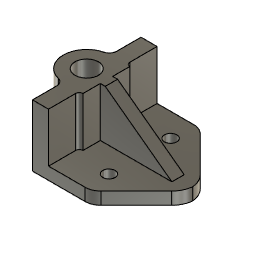
A3 (Autodesk Fusion 360 design; units mm, degrees)
Autodesk Fusion 360 part; units mm, degrees
sketch "Sketch1" plane through (0, 0, 0) normal (0, 0, 1) x (1, 0, 0)
  line L0 (-0.3848, 44) -> (-43, 44)
  line L1 (-43, 44) -> (-43, -44)
  line L2 (-43, -44) -> (-0.3848, -44)
  line L3 (43, 1.8701) -> (43, -1.8701)
  line L4 (37.435, 11.565) -> (8.8076, 40.1924)
  line L5 (37.435, -11.565) -> (8.8076, -40.1924)
  arc A0 (43, -1.8701) -> (37.435, 11.565) centre (24, -1.8701) ccw
  arc A1 (37.435, -11.565) -> (43, 1.8701) centre (24, 1.8701) ccw
  arc A2 (-0.3848, -44) -> (8.8076, -40.1924) centre (-0.3848, -31) ccw
  arc A3 (8.8076, 40.1924) -> (-0.3848, 44) centre (-0.3848, 31) ccw
  point P0 (43, 6)
  point P1 (5, 44)
  point P2 (43, -6)
  point P3 (5, -44)
  dimension "d2" = 88
  dimension "d7" = 19
  dimension "d8" = 19
  dimension "d9" = 13
  dimension "d10" = 13
  constraint horizontal L0
  constraint perpendicular L0 L1
  constraint parallel L0 L2
  constraint parallel L1 L3
  constraint coincident P0 L4
  constraint coincident L3 P0
  constraint tangent L4 A0
  constraint tangent L3 A0
  constraint coincident P2 L5
  constraint coincident L3 P2
  constraint tangent L5 A1
  constraint tangent L3 A1
  constraint coincident P3 L5
  constraint coincident L2 P3
  constraint tangent L5 A2
  constraint tangent L2 A2
  constraint coincident P1 L4
  constraint coincident L0 P1
  constraint tangent L4 A3
  constraint tangent L0 A3
  measures "d2" distance of L0.end L1.end
  measures "d7" radius of A0
  measures "d8" radius of A1
  measures "d9" radius of A2
  measures "d10" radius of A3
extrude "Extrude1" add sketch "Sketch1" along normal blind 10 contours L0 L1 L2 L4 L5 A0 A1 A2 A3 makes body 1
sketch "Sketch3" plane through (0, 0, 10) normal (0, 0, 1) x (-1, 0, 0)
  arc A0 (-37.435, 11.565) -> (-42.9077, 0) centre (-24, -1.8701) ccw
  arc A1 (-42.9077, 0) -> (-37.435, -11.565) centre (-24, 1.8701) ccw
  line L0 (-37.435, -11.565) -> (-8.8076, -40.1924)
  arc A2 (-8.8076, -40.1924) -> (0.3848, -44) centre (0.3848, -31) ccw
  line L1 (0.3848, -44) -> (43, -44)
  line L2 (43, -44) -> (43, 44)
  line L3 (43, 44) -> (0.3848, 44)
  arc A3 (0.3848, 44) -> (-8.8076, 40.1924) centre (0.3848, 31) ccw
  line L4 (-8.8076, 40.1924) -> (-37.435, 11.565)
  line L5 (43, 44) -> (30, 44)
  line L6 (30, -44) -> (43, -44)
  line L7 (27, -19) -> (27, -19)
  line L8 (27, 19) -> (27, 19)
  line L9 (30, -22) -> (30, -44)
  line L10 (30, 44) -> (30, 22)
  arc A4 (30, -22) -> (27, -19) centre (27, -22) ccw
  arc A5 (27, 19) -> (30, 22) centre (27, 22) ccw
  circle A6 centre (43, 0) radius 9.5
  line L11 (43, -44) -> (43, -24.2693)
  line L12 (43, 24.2693) -> (43, 44)
  arc A7 (47.56, -18.4447) -> (47.56, 18.4447) centre (43, 0) ccw
  arc A8 (43, 24.2693) -> (47.56, 18.4447) centre (49, 24.2693) ccw
  arc A9 (47.56, -18.4447) -> (43, -24.2693) centre (49, -24.2693) ccw
  line L13 (27, -5) -> (23, -5)
  line L14 (23, -5) -> (23, 5)
  line L15 (23, 5) -> (27, 5)
  line L16 (27, -19) -> (27, -5)
  line L17 (27, 5) -> (27, 19)
  dimension "d18" = 13
  dimension "d19" = 88
  dimension "d23" = 3
  dimension "d24" = 3
  dimension "d25" = 38
  dimension "d27" = 6
  dimension "d28" = 6
  dimension "d29" = 4
  dimension "d30" = 10
  dimension "d31" = 39
  constraint horizontal L5
  constraint horizontal L6
  constraint vertical L11
  constraint coincident L2.end L3.start
  constraint vertical L16
  constraint vertical L9
  constraint tangent L9 A4
  constraint tangent L10 A5
  constraint midpoint L2 A6.centre
  constraint tangent L12 A8
  constraint tangent A7 A8
  constraint tangent L11 A9
  constraint tangent A7 A9
  constraint horizontal L13
  constraint vertical L14
  constraint horizontal L15
  constraint collinear L16 L17
  measures "d18" distance of L2.end L5.end
  measures "d19" distance of L2.end L1.end
  measures "d23" radius of A4
  measures "d24" radius of A5
  measures "d25" diameter of A7
  measures "d27" radius of A8
  measures "d28" radius of A9
  measures "d29" distance of L13.start L13.end
  measures "d30" distance of L13.start L15.end
  measures "d31" distance of L6 L13
extrude "Extrude2" add sketch "Sketch3" along normal blind 40 separate body contours L1 L2 L3 L5 L6 L9 L10 A4 A5 A6 L11 L12 L13 L14 L15 L16 L17 makes body 2
extrude "Extrude3" add sketch "Sketch3" along normal blind 40 and the other way blind 10 contours L2 A6 A7 A8 A9 bodies 2
sketch "Sketch4" plane through (0, 0, 0) normal (0, 0, 1) x (1, 0, 0)
  line L0 (-43.035, -9.4999) -> (-43.035, 9.4999)
  arc A0 (-43.035, -9.4999) -> (-43.035, 9.4999) centre (-43, 0) ccw
  dimension "d38" = 19
  constraint vertical L0
  measures "d38" diameter of A0
extrude "Extrude4" cut sketch "Sketch4" along normal blind 10 bodies 1
sketch "Sketch5" plane through (0, 0, 0) normal (0, 1, 0) x (1, 0, 0)
  line L0 (-23, -10) -> (31, -10)
  line L1 (31, -10) -> (-23, -50)
  line L2 (-23, -50) -> (-23, -10)
  constraint horizontal L0
  constraint perpendicular L0 L2
extrude "Extrude5" add sketch "Sketch5" along normal mid plane 10 bodies 1 2
sketch "Sketch6" plane through (0, 0, 10) normal (0, 0, 1) x (-1, 0, 0)
  line L0 (-31, 5) -> (27, 5)
  line L1 (27, 5) -> (27, 19)
  arc A0 (27, 19) -> (30, 22) centre (27, 22) ccw
  line L2 (30, 22) -> (30, 44)
  line L3 (30, 44) -> (0.3848, 44)
  arc A1 (0.3848, 44) -> (-8.8076, 40.1924) centre (0.3848, 31) ccw
  line L4 (-8.8076, 40.1924) -> (-37.435, 11.565)
  arc A2 (-37.435, 11.565) -> (-42.9077, 0) centre (-24, -1.8701) ccw
  arc A3 (-42.9077, 0) -> (-37.435, -11.565) centre (-24, 1.8701) ccw
  line L5 (-37.435, -11.565) -> (-8.8076, -40.1924)
  arc A4 (-8.8076, -40.1924) -> (0.3848, -44) centre (0.3848, -31) ccw
  line L6 (0.3848, -44) -> (30, -44)
  line L7 (30, -44) -> (30, -22)
  arc A5 (30, -22) -> (27, -19) centre (27, -22) ccw
  line L8 (27, -19) -> (27, -5)
  line L9 (27, -5) -> (-31, -5)
  line L10 (-31, -5) -> (-31, 5)
  circle A6 centre (0, 25) radius 5
  circle A7 centre (0, -25) radius 5
  dimension "d43" = 10
  dimension "d44" = 20
  dimension "d45" = 10
  measures "d43" diameter of A6
  measures "d44" distance of L0 A6.centre
  measures "d45" diameter of A7
extrude "Extrude6" cut sketch "Sketch6" against normal blind 10 contours A6 | A7 bodies 1
equation "d31 = 20 mm + 19 mm"
